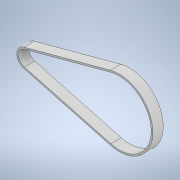
# Autodesk Inventor part: belt
Saved by Autodesk Inventor 2020.3 (Build 243373000, 373)
## iProperties
Created: 2022-01-06
Part Number: belt
Material: Generic
Document SubType Name: Modeling
Designer: Martijn
Density: 1 g/cm^3
Appearance: Default
Author: Martijn
Autodesk Inventor part; units mm, degrees
ref_plane "YZ Plane" through (0, 0, 0) normal (1, 0, 0) x (0, 1, 0)
ref_plane "XZ Plane" through (0, 0, 0) normal (0, 1, 0) x (-1, 0, 0)
ref_plane "XY Plane" through (0, 0, 0) normal (0, 0, 1) x (1, 0, 0)
sketch "Sketch1" plane through (0, 0, 0) normal (0, 0, 1) x (1, 0, 0)
  arc A0 (-1.3223, 4.921) -> (-1.3223, -4.921) centre (0, 0) ccw
  line L0 (-1.3223, 4.921) -> (49.0415, 18.4537)
  line L1 (-1.3223, -4.921) -> (49.0415, -18.4537)
  arc A1 (49.0415, -18.4537) -> (49.0415, 18.4537) centre (54, 0) ccw
  arc A2 (-1.1925, 4.4381) -> (-1.1925, -4.4381) centre (0, 0) ccw
  arc A3 (49.1712, -17.9708) -> (49.1712, 17.9708) centre (54, 0) ccw
  arc A4 (48.9117, -18.9366) -> (48.9117, 18.9366) centre (54, 0) ccw
  arc A5 (-1.452, 5.4039) -> (-1.452, -5.4039) centre (0, 0) ccw
  line L2 (-1.452, 5.4039) -> (48.9117, 18.9366)
  line L3 (49.1712, 17.9708) -> (-1.1925, 4.4381)
  line L4 (-1.1925, -4.4381) -> (49.1712, -17.9708)
  line L5 (48.9117, -18.9366) -> (-1.452, -5.4039)
  line L6 (-21.4363, 0) -> (89.449, 0) projected
  dimension "d0" = 5.0955
  dimension "d1" = 19.1083
  dimension "d9" = 54
  dimension "d10" = 0.5
  dimension "d11" = 0.5
  constraints: 14 point on circle, 12 end point, 12 tangent, 6 centre point, 3 coincident, 2 parallel, 1 point on line
  measures "d0" radius of A0
  measures "d1" radius of A1
  measures "d9" distance of A1.centre A5.centre
  measures "d10" radial gap between concentric circles of A0 A2
  measures "d11" radial gap between concentric circles of A0 A5
extrude "Extrusion1" add sketch "Sketch1" along normal blind 6 contours L0 A1 L6 A3 L3 A2 A0 | A0 L6 A5 L2 A4 A1 L0 | L6 A2 L4 A3 A1 L1 A0 | A0 L1 A1 L6 A4 L5 A5
body "Solid1"
